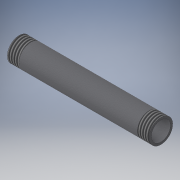
# Autodesk Inventor part: 2 Inch Pipe
Saved by Autodesk Inventor 2019 (Build 230136000, 136)
## iProperties
Created: 2019-08-29
Part Number: 2 Inch Pipe
Material: Iron, Cast
Document SubType Name: Modeling
Designer: Rick Szalay
Density: 7.15 g/cm^3
Appearance: Iron - Cast
Author: Rick Szalay
Autodesk Inventor part; units mm, degrees
ref_plane "YZ Plane" through (0, 0, 0) normal (1, 0, 0) x (0, 1, 0)
ref_plane "XZ Plane" through (0, 0, 0) normal (0, 1, 0) x (-1, 0, 0)
ref_plane "XY Plane" through (0, 0, 0) normal (0, 0, 1) x (1, 0, 0)
sketch "Sketch1" plane through (0, 0, 0) normal (1, 0, 0) x (0, 1, 0)
  circle A0 centre (0, 0) radius 25.4
  dimension "d0" = 50.8
  constraints: 1 centre point, 1 coincident
  measures "d0" diameter of A0
extrude "Extrusion1" add sketch "Sketch1" along normal mid plane 304.8
sketch "Sketch2" plane through (152.4, 0, 0) normal (1, 0, 0) x (0, 0, -1)
  circle A0 centre (0, 0) radius 25.4 projected
  circle A1 centre (0, 0) radius 20.6375
  dimension "d4" = 4.7625
  constraints: 1 centre point
  measures "d4" radial gap between concentric circles of A0 A1
extrude "Extrusion2" cut sketch "Sketch2" against normal through all contours A1
thread "Thread1" size "2-4.5 UNC" class "2A" standard "ANSI Unified Screw Threads" length 25.4
thread "Thread2" size "2-4.5 UNC" class "2A" standard "ANSI Unified Screw Threads" length 25.4
body "Solid1"
